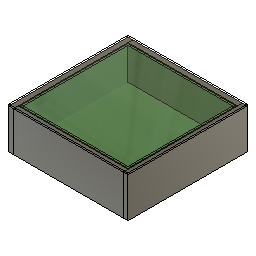
valkyrie_Draw_v6 (Autodesk Fusion 360 design; units mm, degrees)
Autodesk Fusion 360 part; units mm, degrees
sketch "Sketch1" plane through (0, 0, 0) normal (0, 1, 0) x (1, 0, 0) in component "Front"
  line L0 (138, 50) -> (-138, 50)
  line L1 (-138, 50) -> (-138, -50)
  line L2 (-138, -50) -> (138, -50)
  line L3 (138, -50) -> (138, 50)
  line L4 (138, 50) -> (-138, -50) construction
  line L5 (-138, 50) -> (138, -50) construction
  dimension "d1" = 276
  dimension "d6" = 100
  constraint horizontal L0
  constraint perpendicular L0 L1
  constraint parallel L0 L2
  constraint parallel L1 L3
  constraint coincident L4 origin
  constraint coincident L5 origin
  measures "d1" distance of L1.end L2.end
  measures "d6" distance of L0.end L1.end
extrude "Extrude1" add sketch "Sketch1" along normal blind 12 makes body 1 in component "Front"
sketch "Sketch1 (2)" plane through (138, 0, 0) normal (1, 0, 0) x (0, 1, 0) in component "Right Side"
  line L0 (0, 50) -> (0, -50)
  line L1 (0, -50) -> (12, -50)
  line L2 (12, -50) -> (12, 50)
  line L3 (12, 50) -> (0, 50)
  line L4 (12, 50) -> (312, 50)
  line L5 (312, 50) -> (312, -50)
  line L6 (312, -50) -> (12, -50)
  line L7 (12, -50) -> (12, 50)
  dimension "d9" = 300
  dimension "d10" = 100
  constraint horizontal L4
  constraint vertical L5
  constraint horizontal L6
  constraint vertical L7
  constraint coincident L2.end L3.start
  measures "d9" distance of L2.end L4.end
  measures "d10" distance of L2.end L1.end
extrude "Extrude1'" add sketch "Sketch1 (2)" against normal blind 12 separate body contours L2 L4 L5 L6 L7 makes body 2 in component "Right Side"
sketch "Sketch1 (3)" plane through (-138, 0, 0) normal (-1, 0, 0) x (0, -1, 0) in component "Left side"
  line L0 (0, -50) -> (0, 50)
  line L1 (0, 50) -> (-12, 50)
  line L2 (-12, 50) -> (-12, -50)
  line L3 (-12, -50) -> (0, -50)
  line L4 (-12, 50) -> (-312, 50)
  line L5 (-312, 50) -> (-312, -50)
  line L6 (-312, -50) -> (-12, -50)
  line L7 (-12, -50) -> (-12, 50)
  dimension "d13" = 300
  dimension "d14" = 100
  constraint horizontal L4
  constraint vertical L5
  constraint horizontal L6
  constraint vertical L7
  constraint coincident L1.end L2.start
  measures "d13" distance of L1.end L4.end
  measures "d14" distance of L1.end L2.end
extrude "Extrude1''" add sketch "Sketch1 (3)" against normal blind 12 separate body contours L2 L4 L5 L6 L7 makes body 3 in component "Left side"
sketch "Sketch1 (4)" plane through (0, 312, 0) normal (0, 1, 0) x (-1, 0, 0) in component "Back"
  line L0 (-138, 50) -> (-138, -50)
  line L1 (-138, -50) -> (-126, -50)
  line L2 (-126, -50) -> (-126, 50)
  line L3 (-126, 50) -> (-138, 50)
  line L4 (-126, 50) -> (150, 50)
  line L5 (150, 50) -> (150, -50)
  line L6 (150, -50) -> (-126, -50)
  line L7 (-126, -50) -> (-126, 50)
  dimension "d20" = 100
  dimension "d21" = 276
  constraint coincident L2.end L3.start
  constraint vertical L7
  constraint horizontal L4
  constraint vertical L5
  constraint horizontal L6
  measures "d20" distance of L2.end L1.end
  measures "d21" distance of L2.end L4.end
extrude "Extrude1'''" add sketch "Sketch1 (4)" against normal blind 12 separate body contours L2 L4 L5 L6 L7 makes body 4 in component "Back"
sketch "Sketch2" plane through (0, 0, 0) normal (0, 0, 1) x (1, 0, 0) in component "Component5base"
  line L0 (201.5693, 10.5193) -> (477.5693, 10.5193)
  line L1 (477.5693, 10.5193) -> (477.5693, 286.5193)
  line L2 (477.5693, 286.5193) -> (201.5693, 286.5193)
  line L3 (201.5693, 286.5193) -> (201.5693, 10.5193)
  dimension "d38" = 276
  dimension "d39" = 276
  constraint horizontal L0
  constraint vertical L1
  constraint horizontal L2
  constraint vertical L3
  measures "d38" distance of L0.start L0.end
  measures "d39" distance of L0.start L2.end
extrude "Extrude2" add sketch "Sketch2" along normal blind 12 separate body makes body 5 in component "Component5base"
sketch "Sketch1 (5)" plane through (138, 0, 0) normal (-1, 0, 0) x (0, -1, 0) in component "insulation RH side"
  line L0 (-300, -50) -> (0, -50)
  line L1 (0, -50) -> (0, 50)
  line L2 (0, 50) -> (-300, 50)
  line L3 (-300, 50) -> (-300, -50)
  line L4 (-288, 156.4658) -> (-12, 156.4658)
  line L5 (-12, 156.4658) -> (-12, 68.4658)
  line L6 (-12, 68.4658) -> (-288, 68.4658)
  line L7 (-288, 68.4658) -> (-288, 156.4658)
  dimension "d46" = 88
  dimension "d47" = 276
  constraint horizontal L4
  constraint vertical L5
  constraint horizontal L6
  constraint vertical L7
  measures "d46" distance of L4.start L6.end
  measures "d47" distance of L4.start L4.end
extrude "Extrude1''''" add sketch "Sketch1 (5)" along normal blind 2.2 separate body contours L4 L5 L6 L7 makes body 6 in component "insulation RH side"
sketch "Sketch1 (6)" plane through (-138, 0, 0) normal (1, 0, 0) x (0, 1, 0) in component "insulation LH side"
  line L0 (0, 50) -> (0, -50)
  line L1 (0, -50) -> (300, -50)
  line L2 (300, -50) -> (300, 50)
  line L3 (300, 50) -> (0, 50)
  line L4 (18.8584, 118.8317) -> (294.8584, 118.8317)
  line L5 (294.8584, 118.8317) -> (294.8584, 30.8317)
  line L6 (294.8584, 30.8317) -> (18.8584, 30.8317)
  line L7 (18.8584, 30.8317) -> (18.8584, 118.8317)
  dimension "d55" = 276
  dimension "d56" = 88
  constraint horizontal L4
  constraint vertical L5
  constraint horizontal L6
  constraint vertical L7
  measures "d55" distance of L4.start L4.end
  measures "d56" distance of L4.start L6.end
extrude "Extrude1'''''" add sketch "Sketch1 (6)" along normal blind 2.2 separate body contours L3 L4 L5 L7 | L3 L5 L6 L7 makes body 7 in component "insulation LH side"
sketch "Sketch1 (7)" plane through (0, 12, 0) normal (0, 1, 0) x (-1, 0, 0) in component "insulation Front"
  line L0 (-138, 50) -> (-138, -50)
  line L1 (-138, -50) -> (138, -50)
  line L2 (138, -50) -> (138, 50)
  line L3 (138, 50) -> (-138, 50)
  line L4 (-130.6712, 134.0558) -> (140.9288, 134.0558)
  line L5 (140.9288, 134.0558) -> (140.9288, 46.0558)
  line L6 (140.9288, 46.0558) -> (-130.6712, 46.0558)
  line L7 (-130.6712, 46.0558) -> (-130.6712, 134.0558)
  dimension "d63" = 271.6
  dimension "d64" = 88
  constraint horizontal L4
  constraint vertical L5
  constraint horizontal L6
  constraint vertical L7
  measures "d63" distance of L4.start L4.end
  measures "d64" distance of L4.start L6.end
extrude "Extrude1''''''" add sketch "Sketch1 (7)" along normal blind 2.2 separate body contours L2 L3 L4 L5 L6 L7 | L2 L3 L6 L7 makes body 8 in component "insulation Front"
sketch "Sketch1 (8)" plane through (0, 288, 0) normal (0, -1, 0) x (1, 0, 0) in component "insulation Back"
  line L0 (-138, -50) -> (138, -50)
  line L1 (138, -50) -> (138, 50)
  line L2 (138, 50) -> (-138, 50)
  line L3 (-138, 50) -> (-138, -50)
  line L4 (-124.9936, 135.96) -> (146.6064, 135.96)
  line L5 (146.6064, 135.96) -> (146.6064, 47.96)
  line L6 (146.6064, 47.96) -> (-124.9936, 47.96)
  line L7 (-124.9936, 47.96) -> (-124.9936, 135.96)
  dimension "d71" = 271.6
  dimension "d72" = 88
  constraint horizontal L4
  constraint vertical L5
  constraint horizontal L6
  constraint vertical L7
  measures "d71" distance of L4.start L4.end
  measures "d72" distance of L4.start L6.end
extrude "Extrude1'''''''" add sketch "Sketch1 (8)" along normal blind 2.2 separate body contours L1 L2 L6 L7 | L1 L2 L4 L5 L6 L7 makes body 9 in component "insulation Back"
sketch "Sketch1 (9)" plane through (0, 0, -50) normal (0, 0, -1) x (1, 0, 0) in component "insulation base"
  line L0 (-138, -12) -> (-138, -288)
  line L1 (-138, -288) -> (138, -288)
  line L2 (138, -288) -> (138, -12)
  line L3 (138, -12) -> (-138, -12)
  line L4 (-377.3205, -251.0817) -> (-105.7205, -251.0817)
  line L5 (-105.7205, -251.0817) -> (-105.7205, 20.5183)
  line L6 (-105.7205, 20.5183) -> (-377.3205, 20.5183)
  line L7 (-377.3205, 20.5183) -> (-377.3205, -251.0817)
  dimension "d79" = 271.6
  dimension "d80" = 271.6
  constraint horizontal L4
  constraint vertical L5
  constraint horizontal L6
  constraint vertical L7
  measures "d79" distance of L4.start L4.end
  measures "d80" distance of L4.start L6.end
extrude "Extrude1''''''''" add sketch "Sketch1 (9)" along normal blind 2.2 separate body contours L0 L3 L4 L5 | L0 L3 L4 L5 L6 L7 makes body 10 in component "insulation base"
move_body "Move1" bodies 10 to x (1, 0, 0) y (0, 1, 0) z (0, 0, 1) at (-78.9453, 0, 0) in component "insulation base"
sketch "Sketch1 (10)" plane through (0, 14.2, 0) normal (0, 1, 0) x (-1, 0, 0) in component "inner Front"
  line L0 (-135.8, -38) -> (135.8, -38)
  line L1 (135.8, -38) -> (135.8, 50)
  line L2 (135.8, 50) -> (-135.8, 50)
  line L3 (-135.8, 50) -> (-135.8, -38)
  line L4 (-138.9279, 176.9039) -> (132.6721, 176.9039)
  line L5 (132.6721, 176.9039) -> (132.6721, 91.1039)
  line L6 (132.6721, 91.1039) -> (-138.9279, 91.1039)
  line L7 (-138.9279, 91.1039) -> (-138.9279, 176.9039)
  dimension "d91" = 271.6
  dimension "d92" = 85.8
  constraint horizontal L4
  constraint vertical L5
  constraint horizontal L6
  constraint vertical L7
  measures "d91" distance of L4.start L4.end
  measures "d92" distance of L4.start L6.end
extrude "Extrude1'''''''''" add sketch "Sketch1 (10)" along normal blind 4 separate body contours L4 L5 L6 L7 makes body 11 in component "inner Front"
sketch "Sketch1 (11)" plane through (0, 285.8, 0) normal (0, -1, 0) x (1, 0, 0) in component "inner Rear"
  line L0 (-135.8, -38) -> (135.8, -38)
  line L1 (135.8, -38) -> (135.8, 50)
  line L2 (135.8, 50) -> (-135.8, 50)
  line L3 (-135.8, 50) -> (-135.8, -38)
  line L4 (-123.2097, 140.8822) -> (148.3903, 140.8822)
  line L5 (148.3903, 140.8822) -> (148.3903, 56.8822)
  line L6 (148.3903, 56.8822) -> (-123.2097, 56.8822)
  line L7 (-123.2097, 56.8822) -> (-123.2097, 140.8822)
  dimension "d100" = 271.6
  dimension "d101" = 84
  constraint horizontal L4
  constraint vertical L5
  constraint horizontal L6
  constraint vertical L7
  measures "d100" distance of L4.start L4.end
  measures "d101" distance of L4.start L6.end
extrude "Extrude1''''''''''" add sketch "Sketch1 (11)" along normal blind 4 separate body contours L4 L5 L6 L7 makes body 12 in component "inner Rear"
sketch "Sketch2 (2)" plane through (-132.6721, 0, 0) normal (1, 0, 0) x (0, 1, 0) in component "inner Front"
  line L0 (12, 88.9039) -> (288, 88.9039)
  line L1 (288, 88.9039) -> (288, 176.9039)
  line L2 (288, 176.9039) -> (12, 176.9039)
  line L3 (12, 176.9039) -> (12, 88.9039)
sketch "Sketch1 (12)" plane through (-135.8, 0, -126.9039) normal (1, 0, 0) x (0, 1, 0) in component "inner LH Side"
  line L0 (26.7212, 274.2093) -> (290.3212, 274.2093)
  line L1 (290.3212, 274.2093) -> (290.3212, 190.2093)
  line L2 (290.3212, 190.2093) -> (26.7212, 190.2093)
  line L3 (26.7212, 190.2093) -> (26.7212, 274.2093)
  dimension "d108" = 263.6
  dimension "d109" = 84
  constraint horizontal L0
  constraint vertical L1
  constraint horizontal L2
  constraint vertical L3
  measures "d108" distance of L0.start L0.end
  measures "d109" distance of L0.start L2.end
extrude "Extrude1'''''''''''" add sketch "Sketch1 (12)" along normal blind 4 separate body makes body 13 in component "inner LH Side"
sketch "Sketch1 (13)" plane through (135.8, 0, 0) normal (-1, 0, 0) x (0, -1, 0) in component "inner RH Side"
  line L0 (-296.5212, 59.3054) -> (-20.5212, 59.3054)
  line L1 (-20.5212, 59.3054) -> (-20.5212, 147.3054)
  line L2 (-20.5212, 147.3054) -> (-296.5212, 147.3054)
  line L3 (-296.5212, 147.3054) -> (-296.5212, 59.3054)
  line L4 (-303.036, 274.5125) -> (-39.436, 274.5125)
  line L5 (-39.436, 274.5125) -> (-39.436, 190.5125)
  line L6 (-39.436, 190.5125) -> (-303.036, 190.5125)
  line L7 (-303.036, 190.5125) -> (-303.036, 274.5125)
  dimension "d116" = 263.6
  dimension "d117" = 84
  constraint horizontal L4
  constraint vertical L5
  constraint horizontal L6
  constraint vertical L7
  measures "d116" distance of L4.start L4.end
  measures "d117" distance of L4.start L6.end
extrude "Extrude1''''''''''''" add sketch "Sketch1 (13)" along normal blind 4 separate body contours L4 L5 L6 L7 makes body 14 in component "inner RH Side"
sketch "Sketch1 (14)" plane through (0, 0, 61.5054) normal (0, 0, 1) x (-1, 0, 0) in component "inner Base"
  line L0 (135.8, -294.3212) -> (135.8, -22.7212)
  line L1 (135.8, -22.7212) -> (-135.8, -22.7212)
  line L2 (-135.8, -22.7212) -> (-135.8, -294.3212)
  line L3 (-135.8, -294.3212) -> (135.8, -294.3212)
  line L4 (547.6575, -340.5039) -> (280.0575, -340.5039)
  line L5 (280.0575, -340.5039) -> (280.0575, -76.9039)
  line L6 (280.0575, -76.9039) -> (547.6575, -76.9039)
  line L7 (547.6575, -76.9039) -> (547.6575, -340.5039)
  dimension "d124" = 267.6
  dimension "d125" = 263.6
  constraint horizontal L4
  constraint vertical L5
  constraint horizontal L6
  constraint vertical L7
  measures "d124" distance of L4.start L4.end
  measures "d125" distance of L4.start L6.end
extrude "Extrude1'''''''''''''" add sketch "Sketch1 (14)" along normal blind 4 separate body contours L4 L5 L6 L7 makes body 15 in component "inner Base"
sketch "Sketch2 (3)" plane through (0, 0, 147.3054) normal (0, 0, 1) x (-1, 0, 0) in component "Lid"
  line L0 (150, -308.5212) -> (150, -8.5212)
  line L1 (150, -8.5212) -> (138, -8.5212)
  line L2 (138, -8.5212) -> (138, -308.5212)
  line L3 (138, -308.5212) -> (150, -308.5212)
  line L4 (376.0435, -297.3721) -> (76.0435, -297.3721)
  line L5 (76.0435, -297.3721) -> (76.0435, 2.6279)
  line L6 (76.0435, 2.6279) -> (376.0435, 2.6279)
  line L7 (376.0435, 2.6279) -> (376.0435, -297.3721)
  dimension "d132" = 300
  dimension "d133" = 300
  constraint horizontal L4
  constraint vertical L5
  constraint horizontal L6
  constraint vertical L7
  measures "d132" distance of L4.start L4.end
  measures "d133" distance of L4.start L6.end
extrude "Extrude1''''''''''''''" add sketch "Sketch2 (3)" along normal blind 4 separate body contours L0 L1 L2 L4 | L0 L1 L2 L4 L5 L6 L7 makes body 16 in component "Lid"
component "Front" placed x (1, 0, 0) y (0, 1, 0) z (0, 0, 1) at (0, 8.5212, 97.3054)
component "Right Side" placed x (1, 0, 0) y (0, 1, 0) z (0, 0, 1) at (12, -3.4788, 97.3054)
component "Left side" placed x (1, 0, 0) y (0, 1, 0) z (0, 0, 1) at (-12, -3.4788, 97.3054)
component "Back" placed x (1, 0, 0) y (0, 1, 0) z (0, 0, 1) at (12, -3.4788, 97.3054)
component "Component5base" placed x (1, 0, 0) y (0, 1, 0) z (0, 0, 1) at (-339.5693, 10.0019, 47.3054)
component "insulation RH side" placed x (1, 0, 0) y (0, 1, 0) z (0, 0, 1) at (0, 8.5212, -9.1604)
component "insulation LH side" placed x (1, 0, 0) y (0, 1, 0) z (0, 0, 1) at (0, 1.6628, 28.4737)
component "insulation Front" placed x (1, 0, 0) y (0, 1, 0) z (0, 0, 1) at (5.1288, 8.5212, 13.2496)
component "insulation Back" placed x (1, 0, 0) y (0, 1, 0) z (0, 0, 1) at (-10.8064, 8.5212, 11.3454)
component "insulation base" placed x (1, 0, 0) y (0, 1, 0) z (0, 0, 1) at (320.4658, 43.2394, 111.5054)
component "inner Front" placed x (1, 0, 0) y (0, 1, 0) z (0, 0, 1) at (-3.1279, 8.5212, -29.5985)
component "inner Rear" placed x (1, 0, 0) y (0, 1, 0) z (0, 0, 1) at (-12.5903, 8.5212, 6.4232)
component "inner RH Side" placed x (1, 0, 0) y (0, 1, 0) z (0, 0, 1) at (0, -12.7148, -127.2071)
component "inner LH Side" placed x (1, 0, 0) y (0, 1, 0) z (0, 0, 1) at (0, 0, 0)
component "inner Base" placed x (1, 0, 0) y (0, 1, 0) z (0, 0, 1) at (411.8575, -50.1827, 1.8)
component "Lid" placed x (1, 0, 0) y (0, 1, 0) z (0, 0, 1) at (226.0435, 11.1491, 0)
equation "d1 = drawerWidth - ( thicknessMDF * 2 )"
equation "drawerWidth = 300 mm"
equation "drawerHeight = 100 mm"
equation "drawerDepth = 300 mm"
equation "thicknessMDF = 12 mm"
equation "d6 = drawerHeight"
equation "d7 = thicknessMDF"
equation "d9 = drawerDepth"
equation "d10 = drawerHeight"
equation "d11 = -thicknessMDF"
equation "d13 = drawerDepth"
equation "d14 = drawerHeight"
equation "d15 = -thicknessMDF"
equation "d20 = drawerHeight"
equation "d21 = drawerWidth - ( thicknessMDF * 2 )"
equation "d22 = -thicknessMDF"
equation "d38 = drawerWidth - ( thicknessMDF * 2 )"
equation "d39 = drawerDepth - ( thicknessMDF * 2 )"
equation "d40 = thicknessMDF"
equation "d46 = drawerHeight - thicknessMDF"
equation "d47 = drawerDepth - ( 2 * thicknessMDF )"
equation "thicknessInsulation = 2.2 mm"
equation "d49 = thicknessInsulation"
equation "d55 = drawerDepth - ( 2 * thicknessMDF )"
equation "d56 = drawerHeight - thicknessMDF"
equation "d57 = thicknessInsulation"
equation "d63 = drawerWidth - ( 2 * thicknessMDF ) - ( 2 * thicknessInsulation )"
equation "d64 = drawerHeight - thicknessMDF"
equation "d65 = thicknessInsulation"
equation "d71 = drawerWidth - ( 2 * thicknessMDF ) - 2 * thicknessInsulation"
equation "d72 = drawerHeight - thicknessMDF"
equation "d73 = thicknessInsulation"
equation "d79 = drawerWidth - ( 2 * thicknessMDF ) - ( 2 * thicknessInsulation )"
equation "d80 = drawerDepth - ( 2 * thicknessMDF ) - ( 2 * thicknessInsulation )"
equation "d81 = thicknessInsulation"
equation "d91 = drawerWidth - ( 2 * thicknessMDF ) - ( 2 * thicknessInsulation )"
equation "d92 = drawerHeight - thicknessMDF - thicknessInsulation"
equation "d93 = thicknessInnerlining"
equation "thicknessInnerlining = 4 mm"
equation "d100 = drawerWidth - ( 2 * thicknessInsulation + 2 * thicknessMDF )"
equation "d101 = drawerHeight - ( thicknessMDF + thicknessInnerlining )"
equation "d102 = thicknessInnerlining"
equation "d108 = drawerDepth - ( 2 * thicknessMDF + 2 * thicknessInsulation ) - 2 * thicknessInnerlining"
equation "d109 = drawerHeight - ( thicknessMDF + thicknessInnerlining )"
equation "d110 = thicknessInnerlining"
equation "d116 = drawerDepth - ( 2 * thicknessMDF + 2 * thicknessInsulation ) - 2 * thicknessInnerlining"
equation "d117 = drawerHeight - ( thicknessMDF + thicknessInnerlining )"
equation "d118 = thicknessInnerlining"
equation "d124 = drawerWidth - ( 2 * thicknessInsulation + 2 * thicknessMDF + thicknessInnerlining )"
equation "d125 = drawerDepth - ( 2 * thicknessMDF + 2 * thicknessInsulation + 2 * thicknessInnerlining )"
equation "d126 = thicknessInnerlining"
equation "d132 = drawerWidth"
equation "d133 = drawerDepth"
equation "d134 = thicknessInnerlining"
